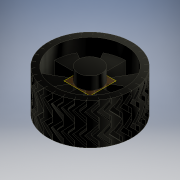
# Autodesk Inventor part: llanta xddd
Saved by Autodesk Inventor 2017 (Build 210142000, 142)
## iProperties
Part Number: llanta xddd
Material: Goma
Document SubType Name: Modeling
Designer: Salvador
Density: 0.93 g/cm^3
Appearance: Gris plomo
Author: Salvador
Autodesk Inventor part; units mm, degrees
ref_plane "YZ Plane" through (0, 0, 0) normal (1, 0, 0) x (0, 1, 0)
ref_plane "XZ Plane" through (0, 0, 0) normal (0, 1, 0) x (-1, 0, 0)
sketch "Boceto1" plane through (0, 0, 0) normal (0, 0, 1) x (1, 0, 0)
  circle A0 centre (0, 0) radius 26.5
  circle A1 centre (0, 0) radius 22.5
  dimension "d0" = 53
  dimension "d1" = 45
  constraints: 2 centre point, 2 coincident
  measures "d0" diameter of A0
  measures "d1" diameter of A1
extrude "Extrusión1" add sketch "Boceto1" along normal blind 26
sketch "Boceto2" plane through (0, 0, 26) normal (0, 0, 1) x (1, 0, 0)
  circle A0 centre (0, 0) radius 7.5
  dimension "d4" = 15
  constraints: 1 centre point, 1 coincident
  measures "d4" diameter of A0
extrude "Extrusión2" add sketch "Boceto2" against normal blind 26
ref_plane "Plano de trabajo1" through (0, 0, 18) normal (0, 0, 1) x (1, 0, 0)
sketch "Boceto3" plane through (0, 0, 18) normal (0, 0, 1) x (1, 0, 0)
  circle A0 centre (0, 0) radius 22.5 projected
  circle A1 centre (0, 0) radius 7.5 projected
  circle A2 centre (0, 0) radius 22.5
  line L0 (-3.75, 6.4952) -> (-11.25, 19.4856)
  line L1 (0, 7.5) -> (0, 22.5)
  circle A3 centre (0, 0) radius 7.5
  dimension "d8" = 30
  dimension "d9" = 15
  dimension "d10" = 0
  constraints: 6 point on circle, 4 end point, 2 centre point, 2 coincident, 1 vertical, 1 vertical alignment
  measures "d8" angle of L0 L1
  measures "d9" diameter of A3
  measures "d10" distance from line of A1.centre L0
extrude "Extrusión3" add sketch "Boceto3" against normal blind 8 contours L1 A1 L0 A0 picked at (-7.1702, 15.8921)
pattern_circular "Patrón circular1" count 6 over 360 about axis through (0, 0, 0) along (0, 0, 1) of "Extrusión3"
ref_plane "Plano de trabajo2" through (13.25, 22.9497, 0) normal (-0.5, -0.866, 0) x (0.866, -0.5, 0)
sketch "Boceto5" plane through (13.25, 22.9497, 0) normal (-0.5, -0.866, 0) x (0.866, -0.5, 0)
  line L0 (0, 0) -> (6.5, 6.5)
  line L1 (6.5, 6.5) -> (0, 13)
  line L2 (7.5, 26) -> (7.5, 0) projected
  line L3 (26.5, 26) -> (-26.5, 26) projected
  line L4 (0, 13) -> (6.5, 19.5)
  line L5 (6.5, 19.5) -> (0, 26)
  line L6 (0, 3.25) -> (3.25, 6.5)
  line L7 (3.25, 6.5) -> (0, 9.75)
  line L8 (0, 16.25) -> (3.25, 19.5)
  line L9 (3.25, 19.5) -> (0, 22.75)
  line L10 (0, 22.75) -> (0, 26)
  line L11 (0, 13) -> (0, 16.25)
  line L12 (0, 0) -> (0, 3.25)
  line L13 (0, 10) -> (3.75, 10) projected
  line L14 (0, 10) -> (0, 13)
  line L15 (0, 9.75) -> (0, 10)
  dimension "d16" = 13
  dimension "d19" = 90
  dimension "d20" = 90
  dimension "d21" = 13
  dimension "d22" = 6.5
  dimension "d23" = 90
  dimension "d24" = 90
  dimension "d25" = 6.8943
  dimension "d26" = 2.2981
  dimension "d27" = 11.4905
  dimension "d28" = 2.2981
  dimension "d29" = 16.25
  constraints: 26 end point, 5 parallel, 1 midpoint, 1 vertical alignment
  measures "d16" distance of L1.end L0.start
  measures "d19" angle of L5 L4
  measures "d20" angle of L1 L0
  measures "d21" distance of L5.end L1.end
  measures "d22" horizontal distance of L0.start L0.end
  measures "d23" angle of L13 L10
  measures "d24" angle of L13 L11
  measures "d25" distance between parallel lines of L9 L1
  measures "d26" distance between parallel lines of L7 L1
  measures "d27" distance between parallel lines of L8 L0
  measures "d28" distance between parallel lines of L6 L0
  measures "d29" distance from line of L7.end L3
extrude "Extrusión4" cut sketch "Boceto5" along normal blind 2
pattern_circular "Patrón circular2" count 30 over 360 about axis through (0, 0, 0) along (0, 0, 1) of "Extrusión4"
sketch "Boceto6" plane through (0, 0, 0) normal (0, 0, -1) x (-1, 0, 0)
  circle A0 centre (0, 0) radius 4.025
  dimension "d35" = 8.05
  constraints: 1 centre point, 1 coincident
  measures "d35" diameter of A0
extrude "Extrusión5" cut sketch "Boceto6" against normal blind 6
